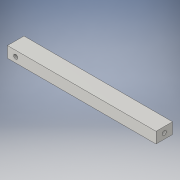
# Autodesk Inventor part: shootFrame
Saved by Autodesk Inventor 2016 (Build 200138000, 138)
## iProperties
Created: 2016-12-21
Part Number: shootFrame
Material: Wood (Birch)
Document SubType Name: Modeling
Designer: Naga
Density: 0.55 g/cm^3
Appearance: White
Author: Naga
Autodesk Inventor part; units mm, degrees
ref_plane "YZ Plane" through (0, 0, 0) normal (1, 0, 0) x (0, 1, 0)
ref_plane "XZ Plane" through (0, 0, 0) normal (0, 1, 0) x (-1, 0, 0)
ref_plane "XY Plane" through (0, 0, 0) normal (0, 0, 1) x (1, 0, 0)
sketch "Sketch1" plane through (0, 0, 0) normal (0, 1, 0) x (-1, 0, 0)
  line L0 (-85.725, 9.525) -> (85.725, 9.525)
  line L1 (85.725, 9.525) -> (85.725, -9.525)
  line L2 (85.725, -9.525) -> (-85.725, -9.525)
  line L3 (-85.725, -9.525) -> (-85.725, 9.525)
  line L4 (-85.725, 9.525) -> (85.725, -9.525) construction
  line L5 (85.725, 9.525) -> (-85.725, -9.525) construction
  point P0 (0, 0)
  dimension "d0" = 171.45
  dimension "d1" = 19.05
  constraints: 12 end point, 2 midpoint, 2 parallel, 1 horizontal, 1 perpendicular
  measures "d0" distance of L1.end L2.end
  measures "d1" distance of L0.end L1.end
extrude "Extrusion1" add sketch "Sketch1" along normal blind 12.7
sketch "Sketch2" plane through (85.725, 0, 9.525) normal (1, 0, 0) x (0, 0, -1)
  line L0 (0, 0) -> (0, 12.7) projected
  line L1 (0, 6.35) -> (19.05, 6.35)
  line L2 (19.05, 0) -> (19.05, 12.7) projected
  circle A0 centre (9.525, 6.35) radius 2.3812
  point P0 (9.525, 0)
  dimension "d4" = 4.7625
  constraints: 3 midpoint, 2 end point, 1 centre point
  measures "d4" diameter of A0
extrude "Extrusion2" cut sketch "Sketch2" against normal blind 12.7
sketch "Sketch3" plane through (-85.725, 0, 9.525) normal (0, 0, 1) x (1, 0, 0)
  line L0 (0, 0) -> (0, 12.7) projected
  line L1 (0, 6.35) -> (9.525, 6.35)
  circle A0 centre (9.525, 6.35) radius 2.3812
  point P0 (85.725, 0)
  dimension "d7" = 9.525
  dimension "d8" = 4.7625
  constraints: 2 end point, 1 centre point, 1 coincident, 1 horizontal, 1 midpoint
  measures "d7" distance of L1.start L1.end
  measures "d8" diameter of A0
extrude "Extrusion3" cut sketch "Sketch3" against normal blind 12.7
body "Solid1"
